Autodesk Fusion 360 part; units mm, degrees
(part 18 of 40)
  spline S39 degree 5 poles (-5.6951, -60.7685) (-5.6979, -60.7993) (-5.7029, -60.8609) (-5.7078, -60.9533) (-5.7097, -61.0766) (-5.7056, -61.231) (-5.6969, -61.3856) (-5.6854, -61.5403) (-5.6723, -61.695) (-5.6583, -61.8498) (-5.6431, -62.0045) (-5.6265, -62.1593) (-5.608, -62.314) (-5.5871, -62.4688) (-5.5641, -62.6235) (-5.539, -62.7782) (-5.5121, -62.9329) (-5.4838, -63.0875) (-5.4542, -63.2421) (-5.4233, -63.3966) (-5.3913, -63.5511) (-5.3579, -63.7055) (-5.3232, -63.8598) (-5.2871, -64.014) (-5.2497, -64.1682) (-5.2109, -64.3222) (-5.1709, -64.4762) (-5.1297, -64.6301) (-5.0873, -64.7839) (-5.0439, -64.9376) (-4.9993, -65.0912) (-4.9536, -65.2447) (-4.9068, -65.398) (-4.8589, -65.5513) (-4.8099, -65.7044) (-4.7599, -65.8574) (-4.7087, -66.0103) (-4.6566, -66.1631) (-4.6035, -66.3158) (-4.5493, -66.4683) (-4.4942, -66.6206) (-4.438, -66.7729) (-4.381, -66.925) (-4.3229, -67.077) (-4.2639, -67.2288) (-4.2039, -67.3804) (-4.143, -67.532) (-4.0812, -67.6833) (-4.0185, -67.8345) (-3.9548, -67.9856) (-3.8903, -68.1365) (-3.8249, -68.2872) (-3.7585, -68.4378) (-3.6913, -68.5882) (-3.6233, -68.7384) (-3.5543, -68.8885) (-3.4846, -69.0384) (-3.4139, -69.1881) (-3.3425, -69.3376) (-3.2701, -69.487) (-3.197, -69.6362) (-3.123, -69.7852) (-3.0482, -69.934) (-2.9726, -70.0826) (-2.8962, -70.2311) (-2.819, -70.3793) (-2.741, -70.5274) (-2.6622, -70.6752) (-2.5826, -70.8229) (-2.5023, -70.9703) (-2.4211, -71.1176) (-2.3556, -71.2352) (-2.3061, -71.3234) (-2.2729, -71.3821) (-2.2563, -71.4115) knots 0 0 0 0 0 0 0.01428571 0.02857143 0.04285714 0.05714286 0.07142857 0.08571429 0.1 0.11428571 0.12857143 0.14285714 0.15714286 0.17142857 0.18571429 0.2 0.21428571 0.22857143 0.24285714 0.25714286 0.27142857 0.28571429 0.3 0.31428571 0.32857143 0.34285714 0.35714286 0.37142857 0.38571429 0.4 0.41428571 0.42857143 0.44285714 0.45714286 0.47142857 0.48571429 0.5 0.51428571 0.52857143 0.54285714 0.55714286 0.57142857 0.58571429 0.6 0.61428571 0.62857143 0.64285714 0.65714286 0.67142857 0.68571429 0.7 0.71428571 0.72857143 0.74285714 0.75714286 0.77142857 0.78571429 0.8 0.81428571 0.82857143 0.84285714 0.85714286 0.87142857 0.88571429 0.9 0.91428571 0.92857143 0.94285714 0.95714286 0.97142857 0.98571429 1 1 1 1 1 1
  line L39 (-5.5428, -59.1442) -> (-5.6951, -60.7685)
  arc A78 (-5.5428, -59.1442) -> (-7.2806, -56.9737) centre (-7.5341, -58.9575) ccw
  arc A79 (-10.6816, -56.435) -> (-7.2806, -56.9737) centre (0, 0) ccw
  arc A80 (-27.5982, -50.3721) -> (-24.5301, -51.9354) centre (0, 0) ccw
  line L40 (24.1948, -56.0345) -> (24.2071, -56.0628) construction
  line L41 (24.2071, -56.0628) -> (24.2308, -56.1198) construction
  line L42 (24.2308, -56.1198) -> (24.264, -56.2062) construction
  line L43 (24.264, -56.2062) -> (24.3039, -56.3229) construction
  line L44 (24.3039, -56.3229) -> (24.3478, -56.4711) construction
  line L45 (24.3478, -56.4711) -> (24.3873, -56.6208) construction
  line L46 (24.3873, -56.6208) -> (24.4241, -56.7714) construction
  line L47 (24.4241, -56.7714) -> (24.4595, -56.9226) construction
  line L48 (24.4595, -56.9226) -> (24.494, -57.0741) construction
  line L49 (24.494, -57.0741) -> (24.5274, -57.226) construction
  line L50 (24.5274, -57.226) -> (24.5594, -57.3783) construction
  line L51 (24.5594, -57.3783) -> (24.5896, -57.5312) construction
  line L52 (24.5896, -57.5312) -> (24.6176, -57.6848) construction
  line L53 (24.6176, -57.6848) -> (24.6435, -57.8391) construction
  line L54 (24.6435, -57.8391) -> (24.6674, -57.994) construction
  line L55 (24.6674, -57.994) -> (24.6897, -58.1494) construction
  line L56 (24.6897, -58.1494) -> (24.7105, -58.3052) construction
  line L57 (24.7105, -58.3052) -> (24.7301, -58.4614) construction
  line L58 (24.7301, -58.4614) -> (24.7485, -58.6179) construction
  line L59 (24.7485, -58.6179) -> (24.7658, -58.7747) construction
  line L60 (24.7658, -58.7747) -> (24.7818, -58.9318) construction
  line L61 (24.7818, -58.9318) -> (24.7965, -59.0893) construction
  line L62 (24.7965, -59.0893) -> (24.8098, -59.2471) construction
  line L63 (24.8098, -59.2471) -> (24.8218, -59.4053) construction
  line L64 (24.8218, -59.4053) -> (24.8325, -59.5638) construction
  line L65 (24.8325, -59.5638) -> (24.842, -59.7226) construction
  line L66 (24.842, -59.7226) -> (24.8504, -59.8817) construction
  line L67 (24.8504, -59.8817) -> (24.8577, -60.0411) construction
  line L68 (24.8577, -60.0411) -> (24.8638, -60.2007) construction
  line L69 (24.8638, -60.2007) -> (24.8689, -60.3605) construction
  line L70 (24.8689, -60.3605) -> (24.8729, -60.5206) construction
  line L71 (24.8729, -60.5206) -> (24.8757, -60.6809) construction
  line L72 (24.8757, -60.6809) -> (24.8776, -60.8415) construction
  line L73 (24.8776, -60.8415) -> (24.8783, -61.0023) construction
  line L74 (24.8783, -61.0023) -> (24.878, -61.1633) construction
  line L75 (24.878, -61.1633) -> (24.8766, -61.3245) construction
  line L76 (24.8766, -61.3245) -> (24.8742, -61.4859) construction
  line L77 (24.8742, -61.4859) -> (24.8708, -61.6475) construction
  line L78 (24.8708, -61.6475) -> (24.8665, -61.8093) construction
  line L79 (24.8665, -61.8093) -> (24.8611, -61.9712) construction
  line L80 (24.8611, -61.9712) -> (24.8548, -62.1334) construction
  line L81 (24.8548, -62.1334) -> (24.8475, -62.2957) construction
  line L82 (24.8475, -62.2957) -> (24.8392, -62.4581) construction
  line L83 (24.8392, -62.4581) -> (24.83, -62.6207) construction
  line L84 (24.83, -62.6207) -> (24.8199, -62.7835) construction
  line L85 (24.8199, -62.7835) -> (24.8088, -62.9464) construction
  line L86 (24.8088, -62.9464) -> (24.7967, -63.1095) construction
  line L87 (24.7967, -63.1095) -> (24.7838, -63.2727) construction
  line L88 (24.7838, -63.2727) -> (24.77, -63.436) construction
  line L89 (24.77, -63.436) -> (24.7552, -63.5995) construction
  line L90 (24.7552, -63.5995) -> (24.7396, -63.7631) construction
  line L91 (24.7396, -63.7631) -> (24.723, -63.9268) construction
  line L92 (24.723, -63.9268) -> (24.7056, -64.0906) construction
  line L93 (24.7056, -64.0906) -> (24.6873, -64.2545) construction
  line L94 (24.6873, -64.2545) -> (24.6681, -64.4185) construction
  line L95 (24.6681, -64.4185) -> (24.648, -64.5826) construction
  line L96 (24.648, -64.5826) -> (24.6271, -64.7468) construction
  line L97 (24.6271, -64.7468) -> (24.6054, -64.9111) construction
  line L98 (24.6054, -64.9111) -> (24.5828, -65.0755) construction
  line L99 (24.5828, -65.0755) -> (24.5593, -65.24) construction
  line L100 (24.5593, -65.24) -> (24.535, -65.4046) construction
  line L101 (24.535, -65.4046) -> (24.5098, -65.5692) construction
  line L102 (24.5098, -65.5692) -> (24.4839, -65.734) construction
  line L103 (24.4839, -65.734) -> (24.4571, -65.8987) construction
  line L104 (24.4571, -65.8987) -> (24.4294, -66.0636) construction
  line L105 (24.4294, -66.0636) -> (24.401, -66.2285) construction
  line L106 (24.401, -66.2285) -> (24.3718, -66.3935) construction
  line L107 (24.3718, -66.3935) -> (24.3417, -66.5585) construction
  line L108 (24.3417, -66.5585) -> (24.3108, -66.7236) construction
  line L109 (24.3108, -66.7236) -> (24.2792, -66.8887) construction
  line L110 (24.2792, -66.8887) -> (24.2532, -67.0208) construction
  line L111 (24.2532, -67.0208) -> (24.2334, -67.1199) construction
  line L112 (24.2334, -67.1199) -> (24.22, -67.186) construction
  line L113 (24.22, -67.186) -> (24.2132, -67.2191) construction
  line L114 (60.7685, -5.6951) -> (60.7993, -5.6979) construction
  line L115 (60.7993, -5.6979) -> (60.8609, -5.7029) construction
  line L116 (60.8609, -5.7029) -> (60.9533, -5.7078) construction
  line L117 (60.9533, -5.7078) -> (61.0766, -5.7097) construction
  line L118 (61.0766, -5.7097) -> (61.231, -5.7056) construction
  line L119 (61.231, -5.7056) -> (61.3856, -5.6969) construction
  line L120 (61.3856, -5.6969) -> (61.5403, -5.6854) construction
  line L121 (61.5403, -5.6854) -> (61.695, -5.6723) construction
  line L122 (61.695, -5.6723) -> (61.8498, -5.6583) construction
  line L123 (61.8498, -5.6583) -> (62.0045, -5.6431) construction
  line L124 (62.0045, -5.6431) -> (62.1593, -5.6265) construction
  line L125 (62.1593, -5.6265) -> (62.314, -5.608) construction
  line L126 (62.314, -5.608) -> (62.4688, -5.5871) construction
  line L127 (62.4688, -5.5871) -> (62.6235, -5.5641) construction
  line L128 (62.6235, -5.5641) -> (62.7782, -5.539) construction
  line L129 (62.7782, -5.539) -> (62.9329, -5.5121) construction
  line L130 (62.9329, -5.5121) -> (63.0875, -5.4838) construction
  line L131 (63.0875, -5.4838) -> (63.2421, -5.4542) construction
  line L132 (63.2421, -5.4542) -> (63.3966, -5.4233) construction
  line L133 (63.3966, -5.4233) -> (63.5511, -5.3913) construction
  line L134 (63.5511, -5.3913) -> (63.7055, -5.3579) construction
  line L135 (63.7055, -5.3579) -> (63.8598, -5.3232) construction
  line L136 (63.8598, -5.3232) -> (64.014, -5.2871) construction
  line L137 (64.014, -5.2871) -> (64.1682, -5.2497) construction
  line L138 (64.1682, -5.2497) -> (64.3222, -5.2109) construction
  line L139 (64.3222, -5.2109) -> (64.4762, -5.1709) construction
  line L140 (64.4762, -5.1709) -> (64.6301, -5.1297) construction
  line L141 (64.6301, -5.1297) -> (64.7839, -5.0873) construction
  line L142 (64.7839, -5.0873) -> (64.9376, -5.0439) construction
  line L143 (64.9376, -5.0439) -> (65.0912, -4.9993) construction
  line L144 (65.0912, -4.9993) -> (65.2447, -4.9536) construction
  line L145 (65.2447, -4.9536) -> (65.398, -4.9068) construction
  line L146 (65.398, -4.9068) -> (65.5513, -4.8589) construction
  line L147 (65.5513, -4.8589) -> (65.7044, -4.8099) construction
  line L148 (65.7044, -4.8099) -> (65.8574, -4.7599) construction
  line L149 (65.8574, -4.7599) -> (66.0103, -4.7087) construction
  line L150 (66.0103, -4.7087) -> (66.1631, -4.6566) construction
  line L151 (66.1631, -4.6566) -> (66.3158, -4.6035) construction
  line L152 (66.3158, -4.6035) -> (66.4683, -4.5493) construction
  line L153 (66.4683, -4.5493) -> (66.6206, -4.4942) construction
  line L154 (66.6206, -4.4942) -> (66.7729, -4.438) construction
  line L155 (66.7729, -4.438) -> (66.925, -4.381) construction
  line L156 (66.925, -4.381) -> (67.077, -4.3229) construction
  line L157 (67.077, -4.3229) -> (67.2288, -4.2639) construction
  line L158 (67.2288, -4.2639) -> (67.3804, -4.2039) construction
  line L159 (67.3804, -4.2039) -> (67.532, -4.143) construction
  line L160 (67.532, -4.143) -> (67.6833, -4.0812) construction
  line L161 (67.6833, -4.0812) -> (67.8345, -4.0185) construction
  line L162 (67.8345, -4.0185) -> (67.9856, -3.9548) construction
  line L163 (67.9856, -3.9548) -> (68.1365, -3.8903) construction
  line L164 (68.1365, -3.8903) -> (68.2872, -3.8249) construction
  line L165 (68.2872, -3.8249) -> (68.4378, -3.7585) construction
  line L166 (68.4378, -3.7585) -> (68.5882, -3.6913) construction
  line L167 (68.5882, -3.6913) -> (68.7384, -3.6233) construction
  line L168 (68.7384, -3.6233) -> (68.8885, -3.5543) construction
  line L169 (68.8885, -3.5543) -> (69.0384, -3.4846) construction
  line L170 (69.0384, -3.4846) -> (69.1881, -3.4139) construction
  line L171 (69.1881, -3.4139) -> (69.3376, -3.3425) construction
  line L172 (69.3376, -3.3425) -> (69.487, -3.2701) construction
  line L173 (69.487, -3.2701) -> (69.6362, -3.197) construction
  line L174 (69.6362, -3.197) -> (69.7852, -3.123) construction
  line L175 (69.7852, -3.123) -> (69.934, -3.0482) construction
  line L176 (69.934, -3.0482) -> (70.0826, -2.9726) construction
  line L177 (70.0826, -2.9726) -> (70.2311, -2.8962) construction
  line L178 (70.2311, -2.8962) -> (70.3793, -2.819) construction
  line L179 (70.3793, -2.819) -> (70.5274, -2.741) construction
  line L180 (70.5274, -2.741) -> (70.6752, -2.6622) construction
  line L181 (70.6752, -2.6622) -> (70.8229, -2.5826) construction
  line L182 (70.8229, -2.5826) -> (70.9703, -2.5023) construction
  line L183 (70.9703, -2.5023) -> (71.1176, -2.4211) construction
  line L184 (71.1176, -2.4211) -> (71.2352, -2.3556) construction
  line L185 (71.2352, -2.3556) -> (71.3234, -2.3061) construction
  line L186 (71.3234, -2.3061) -> (71.3821, -2.2729) construction
  line L187 (71.3821, -2.2729) -> (71.4115, -2.2563) construction
  line L188 (-45.8153, -40.3263) -> (-45.8385, -40.3467) construction
  line L189 (-45.8385, -40.3467) -> (-45.8854, -40.3868) construction
  line L190 (-45.8854, -40.3868) -> (-45.9573, -40.4451) construction
  line L191 (-45.9573, -40.4451) -> (-46.056, -40.5192) construction
  line L192 (-46.056, -40.5192) -> (-46.1833, -40.6066) construction
  line L193 (-46.1833, -40.6066) -> (-46.3135, -40.6904) construction
  line L194 (-46.3135, -40.6904) -> (-46.4454, -40.772) construction
  line L195 (-46.4454, -40.772) -> (-46.5782, -40.8524) construction
  line L196 (-46.5782, -40.8524) -> (-46.7117, -40.932) construction
  line L197 (-46.7117, -40.932) -> (-46.8458, -41.0107) construction
  line L198 (-46.8458, -41.0107) -> (-46.9807, -41.0883) construction
  line L199 (-46.9807, -41.0883) -> (-47.1168, -41.1642) construction
  line L200 (-47.1168, -41.1642) -> (-47.2543, -41.2383) construction
  line L201 (-47.2543, -41.2383) -> (-47.393, -41.3106) construction
  line L202 (-47.393, -41.3106) -> (-47.5329, -41.3813) construction
  line L203 (-47.5329, -41.3813) -> (-47.6738, -41.4504) construction
  line L204 (-47.6738, -41.4504) -> (-47.8156, -41.5184) construction
  line L205 (-47.8156, -41.5184) -> (-47.9581, -41.5853) construction
  line L206 (-47.9581, -41.5853) -> (-48.1012, -41.6512) construction
  line L207 (-48.1012, -41.6512) -> (-48.245, -41.716) construction
  line L208 (-48.245, -41.716) -> (-48.3895, -41.7798) construction
  line L209 (-48.3895, -41.7798) -> (-48.5347, -41.8424) construction
  line L210 (-48.5347, -41.8424) -> (-48.6807, -41.9039) construction
  line L211 (-48.6807, -41.9039) -> (-48.8274, -41.9642) construction
  line L212 (-48.8274, -41.9642) -> (-48.9749, -42.0234) construction
  line L213 (-48.9749, -42.0234) -> (-49.123, -42.0815) construction
  line L214 (-49.123, -42.0815) -> (-49.2717, -42.1386) construction
  line L215 (-49.2717, -42.1386) -> (-49.421, -42.1947) construction
  line L216 (-49.421, -42.1947) -> (-49.5709, -42.2499) construction
  line L217 (-49.5709, -42.2499) -> (-49.7214, -42.3041) construction
  line L218 (-49.7214, -42.3041) -> (-49.8724, -42.3574) construction
  line L219 (-49.8724, -42.3574) -> (-50.024, -42.4097) construction
  line L220 (-50.024, -42.4097) -> (-50.1761, -42.461) construction
  line L221 (-50.1761, -42.461) -> (-50.3288, -42.5114) construction
  line L222 (-50.3288, -42.5114) -> (-50.482, -42.5608) construction
  line L223 (-50.482, -42.5608) -> (-50.6358, -42.6094) construction
  line L224 (-50.6358, -42.6094) -> (-50.79, -42.657) construction
  line L225 (-50.79, -42.657) -> (-50.9447, -42.7037) construction
  line L226 (-50.9447, -42.7037) -> (-51.0999, -42.7495) construction
  line L227 (-51.0999, -42.7495) -> (-51.2556, -42.7945) construction
  line L228 (-51.2556, -42.7945) -> (-51.4118, -42.8386) construction
  line L229 (-51.4118, -42.8386) -> (-51.5684, -42.8818) construction
  line L230 (-51.5684, -42.8818) -> (-51.7255, -42.9241) construction
  line L231 (-51.7255, -42.9241) -> (-51.883, -42.9656) construction
  line L232 (-51.883, -42.9656) -> (-52.0409, -43.0063) construction
  line L233 (-52.0409, -43.0063) -> (-52.1993, -43.0461) construction
  line L234 (-52.1993, -43.0461) -> (-52.3581, -43.085) construction
  line L235 (-52.3581, -43.085) -> (-52.5173, -43.1231) construction
  line L236 (-52.5173, -43.1231) -> (-52.6769, -43.1604) construction
  line L237 (-52.6769, -43.1604) -> (-52.8369, -43.1969) construction
  line L238 (-52.8369, -43.1969) -> (-52.9973, -43.2326) construction
  line L239 (-52.9973, -43.2326) -> (-53.1581, -43.2674) construction
  line L240 (-53.1581, -43.2674) -> (-53.3193, -43.3015) construction
  line L241 (-53.3193, -43.3015) -> (-53.4809, -43.3347) construction
  line L242 (-53.4809, -43.3347) -> (-53.6428, -43.3672) construction
  line L243 (-53.6428, -43.3672) -> (-53.8051, -43.3988) construction
  line L244 (-53.8051, -43.3988) -> (-53.9677, -43.4297) construction
  line L245 (-53.9677, -43.4297) -> (-54.1307, -43.4597) construction
  line L246 (-54.1307, -43.4597) -> (-54.294, -43.489) construction
  line L247 (-54.294, -43.489) -> (-54.4577, -43.5175) construction
  line L248 (-54.4577, -43.5175) -> (-54.6217, -43.5453) construction
  line L249 (-54.6217, -43.5453) -> (-54.7861, -43.5723) construction
  line L250 (-54.7861, -43.5723) -> (-54.9508, -43.5984) construction
  line L251 (-54.9508, -43.5984) -> (-55.1158, -43.6239) construction
  line L252 (-55.1158, -43.6239) -> (-55.2811, -43.6486) construction
  line L253 (-55.2811, -43.6486) -> (-55.4467, -43.6725) construction
  line L254 (-55.4467, -43.6725) -> (-55.6126, -43.6956) construction
  line L255 (-55.6126, -43.6956) -> (-55.7789, -43.718) construction
  line L256 (-55.7789, -43.718) -> (-55.9454, -43.7397) construction
  line L257 (-55.9454, -43.7397) -> (-56.1122, -43.7606) construction
  line L258 (-56.1122, -43.7606) -> (-56.2459, -43.7767) construction
  line L259 (-56.2459, -43.7767) -> (-56.3463, -43.7885) construction
  line L260 (-56.3463, -43.7885) -> (-56.4133, -43.7962) construction
  line L261 (-56.4133, -43.7962) -> (-56.4469, -43.8) construction
  line L262 (45.8153, -40.3263) -> (45.8385, -40.3467) construction
  line L263 (45.8385, -40.3467) -> (45.8854, -40.3868) construction
  line L264 (45.8854, -40.3868) -> (45.9573, -40.4451) construction
  line L265 (45.9573, -40.4451) -> (46.056, -40.5192) construction
  line L266 (46.056, -40.5192) -> (46.1833, -40.6066) construction
  line L267 (46.1833, -40.6066) -> (46.3135, -40.6904) construction
  line L268 (46.3135, -40.6904) -> (46.4454, -40.772) construction
  line L269 (46.4454, -40.772) -> (46.5782, -40.8524) construction
  line L270 (46.5782, -40.8524) -> (46.7117, -40.932) construction
  line L271 (46.7117, -40.932) -> (46.8458, -41.0107) construction
  line L272 (46.8458, -41.0107) -> (46.9807, -41.0883) construction
  line L273 (46.9807, -41.0883) -> (47.1168, -41.1642) construction
  line L274 (47.1168, -41.1642) -> (47.2543, -41.2383) construction
  line L275 (47.2543, -41.2383) -> (47.393, -41.3106) construction
  line L276 (47.393, -41.3106) -> (47.5329, -41.3813) construction
  line L277 (47.5329, -41.3813) -> (47.6738, -41.4504) construction
  line L278 (47.6738, -41.4504) -> (47.8156, -41.5184) construction
  line L279 (47.8156, -41.5184) -> (47.9581, -41.5853) construction
  line L280 (47.9581, -41.5853) -> (48.1012, -41.6512) construction
  line L281 (48.1012, -41.6512) -> (48.245, -41.716) construction
  line L282 (48.245, -41.716) -> (48.3895, -41.7798) construction
  line L283 (48.3895, -41.7798) -> (48.5347, -41.8424) construction
  line L284 (48.5347, -41.8424) -> (48.6807, -41.9039) construction
  line L285 (48.6807, -41.9039) -> (48.8274, -41.9642) construction
  line L286 (48.8274, -41.9642) -> (48.9749, -42.0234) construction
  line L287 (48.9749, -42.0234) -> (49.123, -42.0815) construction
  line L288 (49.123, -42.0815) -> (49.2717, -42.1386) construction
  line L289 (49.2717, -42.1386) -> (49.421, -42.1947) construction
  line L290 (49.421, -42.1947) -> (49.5709, -42.2499) construction
  line L291 (49.5709, -42.2499) -> (49.7214, -42.3041) construction
  line L292 (49.7214, -42.3041) -> (49.8724, -42.3574) construction
  line L293 (49.8724, -42.3574) -> (50.024, -42.4097) construction
  line L294 (50.024, -42.4097) -> (50.1761, -42.461) construction
  line L295 (50.1761, -42.461) -> (50.3288, -42.5114) construction
  line L296 (50.3288, -42.5114) -> (50.482, -42.5608) construction
  line L297 (50.482, -42.5608) -> (50.6358, -42.6094) construction
  line L298 (50.6358, -42.6094) -> (50.79, -42.657) construction
  line L299 (50.79, -42.657) -> (50.9447, -42.7037) construction
  line L300 (50.9447, -42.7037) -> (51.0999, -42.7495) construction
  line L301 (51.0999, -42.7495) -> (51.2556, -42.7945) construction
  line L302 (51.2556, -42.7945) -> (51.4118, -42.8386) construction
  line L303 (51.4118, -42.8386) -> (51.5684, -42.8818) construction
  line L304 (51.5684, -42.8818) -> (51.7255, -42.9241) construction
  line L305 (51.7255, -42.9241) -> (51.883, -42.9656) construction
  line L306 (51.883, -42.9656) -> (52.0409, -43.0063) construction
  line L307 (52.0409, -43.0063) -> (52.1993, -43.0461) construction
  line L308 (52.1993, -43.0461) -> (52.3581, -43.085) construction
  line L309 (52.3581, -43.085) -> (52.5173, -43.1231) construction
  line L310 (52.5173, -43.1231) -> (52.6769, -43.1604) construction
  line L311 (52.6769, -43.1604) -> (52.8369, -43.1969) construction
  line L312 (52.8369, -43.1969) -> (52.9973, -43.2326) construction
  line L313 (52.9973, -43.2326) -> (53.1581, -43.2674) construction
  line L314 (53.1581, -43.2674) -> (53.3193, -43.3015) construction
  line L315 (53.3193, -43.3015) -> (53.4809, -43.3347) construction
  line L316 (53.4809, -43.3347) -> (53.6428, -43.3672) construction
  line L317 (53.6428, -43.3672) -> (53.8051, -43.3988) construction
  line L318 (53.8051, -43.3988) -> (53.9677, -43.4297) construction
  line L319 (53.9677, -43.4297) -> (54.1307, -43.4597) construction
  line L320 (54.1307, -43.4597) -> (54.294, -43.489) construction
  line L321 (54.294, -43.489) -> (54.4577, -43.5175) construction
  line L322 (54.4577, -43.5175) -> (54.6217, -43.5453) construction
  line L323 (54.6217, -43.5453) -> (54.7861, -43.5723) construction
  line L324 (54.7861, -43.5723) -> (54.9508, -43.5984) construction
  line L325 (54.9508, -43.5984) -> (55.1158, -43.6239) construction
  line L326 (55.1158, -43.6239) -> (55.2811, -43.6486) construction
  line L327 (55.2811, -43.6486) -> (55.4467, -43.6725) construction
  line L328 (55.4467, -43.6725) -> (55.6126, -43.6956) construction
  line L329 (55.6126, -43.6956) -> (55.7789, -43.718) construction
  line L330 (55.7789, -43.718) -> (55.9454, -43.7397) construction
  line L331 (55.9454, -43.7397) -> (56.1122, -43.7606) construction
  line L332 (56.1122, -43.7606) -> (56.2459, -43.7767) construction
  line L333 (56.2459, -43.7767) -> (56.3463, -43.7885) construction
  line L334 (56.3463, -43.7885) -> (56.4133, -43.7962) construction
  line L335 (56.4133, -43.7962) -> (56.4469, -43.8) construction
  line L336 (31.1115, -52.5103) -> (31.1272, -52.5368) construction
  line L337 (31.1272, -52.5368) -> (31.1594, -52.5895) construction
  line L338 (31.1594, -52.5895) -> (31.2097, -52.6672) construction
  line L339 (31.2097, -52.6672) -> (31.2807, -52.7681) construction
  line L340 (31.2807, -52.7681) -> (31.3748, -52.8906) construction
  line L341 (31.3748, -52.8906) -> (31.4727, -53.0106) construction
  line L342 (31.4727, -53.0106) -> (31.5729, -53.1289) construction
  line L343 (31.5729, -53.1289) -> (31.6744, -53.2464) construction
  line L344 (31.6744, -53.2464) -> (31.7767, -53.3634) construction
  line L345 (31.7767, -53.3634) -> (31.88, -53.4797) construction
  line L346 (31.88, -53.4797) -> (31.9844, -53.5951) construction
  line L347 (31.9844, -53.5951) -> (32.0903, -53.7094) construction
  line L348 (32.0903, -53.7094) -> (32.1981, -53.8224) construction
  line L349 (32.1981, -53.8224) -> (32.3077, -53.934) construction
  line L350 (32.3077, -53.934) -> (32.419, -54.0444) construction
  line L351 (32.419, -54.0444) -> (32.5316, -54.1537) construction
  line L352 (32.5316, -54.1537) -> (32.6455, -54.2622) construction
  line L353 (32.6455, -54.2622) -> (32.7603, -54.3698) construction
  line L354 (32.7603, -54.3698) -> (32.876, -54.4767) construction
  line L355 (32.876, -54.4767) -> (32.9927, -54.5828) construction
  line L356 (32.9927, -54.5828) -> (33.1105, -54.6881) construction
  line L357 (33.1105, -54.6881) -> (33.2292, -54.7926) construction
  line L358 (33.2292, -54.7926) -> (33.3491, -54.8961) construction
  line L359 (33.3491, -54.8961) -> (33.47, -54.9988) construction
  line L360 (33.47, -54.9988) -> (33.5919, -55.1007) construction
  line L361 (33.5919, -55.1007) -> (33.7148, -55.2017) construction
  line L362 (33.7148, -55.2017) -> (33.8386, -55.302) construction
  line L363 (33.8386, -55.302) -> (33.9633, -55.4015) construction
  line L364 (33.9633, -55.4015) -> (34.0888, -55.5003) construction
  line L365 (34.0888, -55.5003) -> (34.2151, -55.5984) construction
  line L366 (34.2151, -55.5984) -> (34.3423, -55.6957) construction
  line L367 (34.3423, -55.6957) -> (34.4703, -55.7923) construction
  line L368 (34.4703, -55.7923) -> (34.5991, -55.8881) construction
  line L369 (34.5991, -55.8881) -> (34.7288, -55.9832) construction
  line L370 (34.7288, -55.9832) -> (34.8592, -56.0776) construction
  line L371 (34.8592, -56.0776) -> (34.9905, -56.1712) construction
  line L372 (34.9905, -56.1712) -> (35.1224, -56.2642) construction
  line L373 (35.1224, -56.2642) -> (35.2552, -56.3564) construction
  line L374 (35.2552, -56.3564) -> (35.3886, -56.448) construction
  line L375 (35.3886, -56.448) -> (35.5228, -56.5388) construction
  line L376 (35.5228, -56.5388) -> (35.6577, -56.629) construction
  line L377 (35.6577, -56.629) -> (35.7933, -56.7185) construction
  line L378 (35.7933, -56.7185) -> (35.9295, -56.8073) construction
  line L379 (35.9295, -56.8073) -> (36.0665, -56.8955) construction
  line L380 (36.0665, -56.8955) -> (36.2042, -56.9829) construction
  line L381 (36.2042, -56.9829) -> (36.3425, -57.0697) construction
  line L382 (36.3425, -57.0697) -> (36.4815, -57.1558) construction
  line L383 (36.4815, -57.1558) -> (36.6211, -57.2413) construction
  line L384 (36.6211, -57.2413) -> (36.7614, -57.3261) construction
  line L385 (36.7614, -57.3261) -> (36.9023, -57.4102) construction
  line L386 (36.9023, -57.4102) -> (37.0438, -57.4937) construction
  line L387 (37.0438, -57.4937) -> (37.186, -57.5765) construction
  line L388 (37.186, -57.5765) -> (37.3288, -57.6587) construction
  line L389 (37.3288, -57.6587) -> (37.4721, -57.7403) construction
  line L390 (37.4721, -57.7403) -> (37.6161, -57.8212) construction
  line L391 (37.6161, -57.8212) -> (37.7607, -57.9014) construction
  line L392 (37.7607, -57.9014) -> (37.9058, -57.981) construction
  line L393 (37.9058, -57.981) -> (38.0515, -58.06) construction
  line L394 (38.0515, -58.06) -> (38.1978, -58.1383) construction
  line L395 (38.1978, -58.1383) -> (38.3447, -58.216) construction
  line L396 (38.3447, -58.216) -> (38.4921, -58.2931) construction
  line L397 (38.4921, -58.2931) -> (38.6401, -58.3695) construction
  line L398 (38.6401, -58.3695) -> (38.7886, -58.4453) construction
  line L399 (38.7886, -58.4453) -> (38.9377, -58.5205) construction
  line L400 (38.9377, -58.5205) -> (39.0873, -58.595) construction
  line L401 (39.0873, -58.595) -> (39.2374, -58.669) construction
  line L402 (39.2374, -58.669) -> (39.3881, -58.7423) construction
  line L403 (39.3881, -58.7423) -> (39.5393, -58.8149) construction
  line L404 (39.5393, -58.8149) -> (39.6909, -58.887) construction
  line L405 (39.6909, -58.887) -> (39.8431, -58.9584) construction
  line L406 (39.8431, -58.9584) -> (39.9653, -59.0151) construction
  line L407 (39.9653, -59.0151) -> (40.0572, -59.0573) construction
  line L408 (40.0572, -59.0573) -> (40.1185, -59.0853) construction
  line L409 (40.1185, -59.0853) -> (40.1492, -59.0993) construction
  line L410 (5.6951, -60.7685) -> (5.6979, -60.7993) construction
  line L411 (5.6979, -60.7993) -> (5.7029, -60.8609) construction
  line L412 (5.7029, -60.8609) -> (5.7078, -60.9533) construction
  line L413 (5.7078, -60.9533) -> (5.7097, -61.0766) construction
  line L414 (5.7097, -61.0766) -> (5.7056, -61.231) construction
  line L415 (5.7056, -61.231) -> (5.6969, -61.3856) construction
  line L416 (5.6969, -61.3856) -> (5.6854, -61.5403) construction
  line L417 (5.6854, -61.5403) -> (5.6723, -61.695) construction
  line L418 (5.6723, -61.695) -> (5.6583, -61.8498) construction
  line L419 (5.6583, -61.8498) -> (5.6431, -62.0045) construction
  line L420 (5.6431, -62.0045) -> (5.6265, -62.1593) construction
  line L421 (5.6265, -62.1593) -> (5.608, -62.314) construction
  line L422 (5.608, -62.314) -> (5.5871, -62.4688) construction
  line L423 (5.5871, -62.4688) -> (5.5641, -62.6235) construction
  line L424 (5.5641, -62.6235) -> (5.539, -62.7782) construction
  line L425 (5.539, -62.7782) -> (5.5121, -62.9329) construction
  line L426 (5.5121, -62.9329) -> (5.4838, -63.0875) construction
  line L427 (5.4838, -63.0875) -> (5.4542, -63.2421) construction
  line L428 (5.4542, -63.2421) -> (5.4233, -63.3966) construction
  line L429 (5.4233, -63.3966) -> (5.3913, -63.5511) construction
  line L430 (5.3913, -63.5511) -> (5.3579, -63.7055) construction
  line L431 (5.3579, -63.7055) -> (5.3232, -63.8598) construction
  line L432 (5.3232, -63.8598) -> (5.2871, -64.014) construction
  line L433 (5.2871, -64.014) -> (5.2497, -64.1682) construction
  line L434 (5.2497, -64.1682) -> (5.2109, -64.3222) construction
  line L435 (5.2109, -64.3222) -> (5.1709, -64.4762) construction
  line L436 (5.1709, -64.4762) -> (5.1297, -64.6301) construction
  line L437 (5.1297, -64.6301) -> (5.0873, -64.7839) construction
  line L438 (5.0873, -64.7839) -> (5.0439, -64.9376) construction
  line L439 (5.0439, -64.9376) -> (4.9993, -65.0912) construction
  line L440 (4.9993, -65.0912) -> (4.9536, -65.2447) construction
  line L441 (4.9536, -65.2447) -> (4.9068, -65.398) construction
  line L442 (4.9068, -65.398) -> (4.8589, -65.5513) construction
  line L443 (4.8589, -65.5513) -> (4.8099, -65.7044) construction
  line L444 (4.8099, -65.7044) -> (4.7599, -65.8574) construction
  line L445 (4.7599, -65.8574) -> (4.7087, -66.0103) construction
  line L446 (4.7087, -66.0103) -> (4.6566, -66.1631) construction
  line L447 (4.6566, -66.1631) -> (4.6035, -66.3158) construction
  line L448 (4.6035, -66.3158) -> (4.5493, -66.4683) construction
  line L449 (4.5493, -66.4683) -> (4.4942, -66.6206) construction
  line L450 (4.4942, -66.6206) -> (4.438, -66.7729) construction
  line L451 (4.438, -66.7729) -> (4.381, -66.925) construction
  line L452 (4.381, -66.925) -> (4.3229, -67.077) construction
  line L453 (4.3229, -67.077) -> (4.2639, -67.2288) construction
  line L454 (4.2639, -67.2288) -> (4.2039, -67.3804) construction
  line L455 (4.2039, -67.3804) -> (4.143, -67.532) construction
  line L456 (4.143, -67.532) -> (4.0812, -67.6833) construction
  line L457 (4.0812, -67.6833) -> (4.0185, -67.8345) construction
  line L458 (4.0185, -67.8345) -> (3.9548, -67.9856) construction
  line L459 (3.9548, -67.9856) -> (3.8903, -68.1365) construction
  line L460 (3.8903, -68.1365) -> (3.8249, -68.2872) construction
  line L461 (3.8249, -68.2872) -> (3.7585, -68.4378) construction
  line L462 (3.7585, -68.4378) -> (3.6913, -68.5882) construction
  line L463 (3.6913, -68.5882) -> (3.6233, -68.7384) construction
  line L464 (3.6233, -68.7384) -> (3.5543, -68.8885) construction
  line L465 (3.5543, -68.8885) -> (3.4846, -69.0384) construction
  line L466 (3.4846, -69.0384) -> (3.4139, -69.1881) construction
  line L467 (3.4139, -69.1881) -> (3.3425, -69.3376) construction
  line L468 (3.3425, -69.3376) -> (3.2701, -69.487) construction
  line L469 (3.2701, -69.487) -> (3.197, -69.6362) construction
  line L470 (3.197, -69.6362) -> (3.123, -69.7852) construction
  line L471 (3.123, -69.7852) -> (3.0482, -69.934) construction
  line L472 (3.0482, -69.934) -> (2.9726, -70.0826) construction
  line L473 (2.9726, -70.0826) -> (2.8962, -70.2311) construction
  line L474 (2.8962, -70.2311) -> (2.819, -70.3793) construction
  line L475 (2.819, -70.3793) -> (2.741, -70.5274) construction
  line L476 (2.741, -70.5274) -> (2.6622, -70.6752) construction
  line L477 (2.6622, -70.6752) -> (2.5826, -70.8229) construction
  line L478 (2.5826, -70.8229) -> (2.5023, -70.9703) construction
  line L479 (2.5023, -70.9703) -> (2.4211, -71.1176) construction
  line L480 (2.4211, -71.1176) -> (2.3556, -71.2352) construction
  line L481 (2.3556, -71.2352) -> (2.3061, -71.3234) construction
  line L482 (2.3061, -71.3234) -> (2.2729, -71.3821) construction
  line L483 (2.2729, -71.3821) -> (2.2563, -71.4115) construction
  line L484 (-13.3622, 59.5542) -> (-13.369, 59.5843) construction
  line L485 (-13.369, 59.5843) -> (-13.3833, 59.6444) construction
  line L486 (-13.3833, 59.6444) -> (-13.4071, 59.7338) construction
  line L487 (-13.4071, 59.7338) -> (-13.4435, 59.8517) construction
  line L488 (-13.4435, 59.8517) -> (-13.4951, 59.9973) construction
  line L489 (-13.4951, 59.9973) -> (-13.5511, 60.1416) construction
  line L490 (-13.5511, 60.1416) -> (-13.6099, 60.2852) construction
  line L491 (-13.6099, 60.2852) -> (-13.6701, 60.4283) construction
  line L492 (-13.6701, 60.4283) -> (-13.7313, 60.5711) construction
  line L493 (-13.7313, 60.5711) -> (-13.7935, 60.7136) construction
  line L494 (-13.7935, 60.7136) -> (-13.8571, 60.8557) construction
  line L495 (-13.8571, 60.8557) -> (-13.9226, 60.9971) construction
  line L496 (-13.9226, 60.9971) -> (-13.9902, 61.1379) construction
  line L497 (-13.9902, 61.1379) -> (-14.06, 61.2779) construction
  line L498 (-14.06, 61.2779) -> (-14.1316, 61.4173) construction
  line L499 (-14.1316, 61.4173) -> (-14.205, 61.5561) construction
  line L500 (-14.205, 61.5561) -> (-14.2797, 61.6944) construction
  line L501 (-14.2797, 61.6944) -> (-14.3557, 61.8322) construction
  line L502 (-14.3557, 61.8322) -> (-14.4327, 61.9697) construction
  line L503 (-14.4327, 61.9697) -> (-14.5109, 62.1067) construction
  line L504 (-14.5109, 62.1067) -> (-14.5904, 62.2432) construction
  line L505 (-14.5904, 62.2432) -> (-14.6711, 62.3792) construction
  line L506 (-14.6711, 62.3792) -> (-14.753, 62.5148) construction
  line L507 (-14.753, 62.5148) -> (-14.8363, 62.6498) construction
  line L508 (-14.8363, 62.6498) -> (-14.9208, 62.7843) construction
  line L509 (-14.9208, 62.7843) -> (-15.0064, 62.9184) construction
  line L510 (-15.0064, 62.9184) -> (-15.0932, 63.052) construction
  line L511 (-15.0932, 63.052) -> (-15.181, 63.1852) construction
  line L512 (-15.181, 63.1852) -> (-15.2698, 63.318) construction
  line L513 (-15.2698, 63.318) -> (-15.3597, 63.4503) construction
  line L514 (-15.3597, 63.4503) -> (-15.4506, 63.5821) construction
  line L515 (-15.4506, 63.5821) -> (-15.5425, 63.7135) construction
  line L516 (-15.5425, 63.7135) -> (-15.6354, 63.8445) construction
  line L517 (-15.6354, 63.8445) -> (-15.7293, 63.975) construction
  line L518 (-15.7293, 63.975) -> (-15.8242, 64.105) construction
  line L519 (-15.8242, 64.105) -> (-15.92, 64.2346) construction
  line L520 (-15.92, 64.2346) -> (-16.0168, 64.3638) construction
  line L521 (-16.0168, 64.3638) -> (-16.1146, 64.4926) construction
  line L522 (-16.1146, 64.4926) -> (-16.2132, 64.6209) construction
  line L523 (-16.2132, 64.6209) -> (-16.3127, 64.7488) construction
  line L524 (-16.3127, 64.7488) -> (-16.4131, 64.8762) construction
  line L525 (-16.4131, 64.8762) -> (-16.5144, 65.0032) construction
  line L526 (-16.5144, 65.0032) -> (-16.6166, 65.1298) construction
  line L527 (-16.6166, 65.1298) -> (-16.7196, 65.256) construction
  line L528 (-16.7196, 65.256) -> (-16.8235, 65.3817) construction
  line L529 (-16.8235, 65.3817) -> (-16.9283, 65.507) construction
  line L530 (-16.9283, 65.507) -> (-17.0338, 65.6318) construction
  line L531 (-17.0338, 65.6318) -> (-17.1402, 65.7562) construction
  line L532 (-17.1402, 65.7562) -> (-17.2474, 65.8802) construction
  line L533 (-17.2474, 65.8802) -> (-17.3555, 66.0038) construction
  line L534 (-17.3555, 66.0038) -> (-17.4643, 66.1269) construction
  line L535 (-17.4643, 66.1269) -> (-17.5739, 66.2497) construction
  line L536 (-17.5739, 66.2497) -> (-17.6842, 66.3719) construction
  line L537 (-17.6842, 66.3719) -> (-17.7954, 66.4938) construction
  line L538 (-17.7954, 66.4938) -> (-17.9073, 66.6152) construction
  line L539 (-17.9073, 66.6152) -> (-18.02, 66.7362) construction
  line L540 (-18.02, 66.7362) -> (-18.1335, 66.8568) construction
  line L541 (-18.1335, 66.8568) -> (-18.2477, 66.9769) construction
  line L542 (-18.2477, 66.9769) -> (-18.3626, 67.0966) construction
  line L543 (-18.3626, 67.0966) -> (-18.4782, 67.2159) construction
  line L544 (-18.4782, 67.2159) -> (-18.5946, 67.3347) construction
  line L545 (-18.5946, 67.3347) -> (-18.7118, 67.4531) construction
  line L546 (-18.7118, 67.4531) -> (-18.8296, 67.5711) construction
  line L547 (-18.8296, 67.5711) -> (-18.9481, 67.6887) construction
  line L548 (-18.9481, 67.6887) -> (-19.0674, 67.8058) construction
  line L549 (-19.0674, 67.8058) -> (-19.1873, 67.9225) construction
  line L550 (-19.1873, 67.9225) -> (-19.3079, 68.0388) construction
  line L551 (-19.3079, 68.0388) -> (-19.4293, 68.1546) construction
  line L552 (-19.4293, 68.1546) -> (-19.5512, 68.27) construction
  line L553 (-19.5512, 68.27) -> (-19.6739, 68.385) construction
  line L554 (-19.6739, 68.385) -> (-19.7726, 68.4767) construction
  line L555 (-19.7726, 68.4767) -> (-19.8469, 68.5452) construction
  line L556 (-19.8469, 68.5452) -> (-19.8966, 68.5908) construction
  line L557 (-19.8966, 68.5908) -> (-19.9215, 68.6136) construction
  line L558 (24.1948, 56.0345) -> (24.2071, 56.0628) construction
  line L559 (24.2071, 56.0628) -> (24.2308, 56.1198) construction
  line L560 (24.2308, 56.1198) -> (24.264, 56.2062) construction
  line L561 (24.264, 56.2062) -> (24.3039, 56.3229) construction
  line L562 (24.3039, 56.3229) -> (24.3478, 56.4711) construction
  line L563 (24.3478, 56.4711) -> (24.3873, 56.6208) construction
  line L564 (24.3873, 56.6208) -> (24.4241, 56.7714) construction
  line L565 (24.4241, 56.7714) -> (24.4595, 56.9226) construction
  line L566 (24.4595, 56.9226) -> (24.494, 57.0741) construction
  line L567 (24.494, 57.0741) -> (24.5274, 57.226) construction
  line L568 (24.5274, 57.226) -> (24.5594, 57.3783) construction
  line L569 (24.5594, 57.3783) -> (24.5896, 57.5312) construction
  line L570 (24.5896, 57.5312) -> (24.6176, 57.6848) construction
  line L571 (24.6176, 57.6848) -> (24.6435, 57.8391) construction
  line L572 (24.6435, 57.8391) -> (24.6674, 57.994) construction
  line L573 (24.6674, 57.994) -> (24.6897, 58.1494) construction
  line L574 (24.6897, 58.1494) -> (24.7105, 58.3052) construction
  line L575 (24.7105, 58.3052) -> (24.7301, 58.4614) construction
  line L576 (24.7301, 58.4614) -> (24.7485, 58.6179) construction
  line L577 (24.7485, 58.6179) -> (24.7658, 58.7747) construction
  line L578 (24.7658, 58.7747) -> (24.7818, 58.9318) construction
  line L579 (24.7818, 58.9318) -> (24.7965, 59.0893) construction
  line L580 (24.7965, 59.0893) -> (24.8098, 59.2471) construction
  line L581 (24.8098, 59.2471) -> (24.8218, 59.4053) construction
  line L582 (24.8218, 59.4053) -> (24.8325, 59.5638) construction
  line L583 (24.8325, 59.5638) -> (24.842, 59.7226) construction
  line L584 (24.842, 59.7226) -> (24.8504, 59.8817) construction
  line L585 (24.8504, 59.8817) -> (24.8577, 60.0411) construction
  line L586 (24.8577, 60.0411) -> (24.8638, 60.2007) construction
  line L587 (24.8638, 60.2007) -> (24.8689, 60.3605) construction
  line L588 (24.8689, 60.3605) -> (24.8729, 60.5206) construction
  line L589 (24.8729, 60.5206) -> (24.8757, 60.6809) construction
  line L590 (24.8757, 60.6809) -> (24.8776, 60.8415) construction
  line L591 (24.8776, 60.8415) -> (24.8783, 61.0023) construction
  line L592 (24.8783, 61.0023) -> (24.878, 61.1633) construction
  line L593 (24.878, 61.1633) -> (24.8766, 61.3245) construction
  line L594 (24.8766, 61.3245) -> (24.8742, 61.4859) construction
  line L595 (24.8742, 61.4859) -> (24.8708, 61.6475) construction
  line L596 (24.8708, 61.6475) -> (24.8665, 61.8093) construction
  line L597 (24.8665, 61.8093) -> (24.8611, 61.9712) construction
  line L598 (24.8611, 61.9712) -> (24.8548, 62.1334) construction
  line L599 (24.8548, 62.1334) -> (24.8475, 62.2957) construction
  line L600 (24.8475, 62.2957) -> (24.8392, 62.4581) construction
  line L601 (24.8392, 62.4581) -> (24.83, 62.6207) construction
  line L602 (24.83, 62.6207) -> (24.8199, 62.7835) construction
  line L603 (24.8199, 62.7835) -> (24.8088, 62.9464) construction
  line L604 (24.8088, 62.9464) -> (24.7967, 63.1095) construction
  line L605 (24.7967, 63.1095) -> (24.7838, 63.2727) construction
  line L606 (24.7838, 63.2727) -> (24.77, 63.436) construction
  line L607 (24.77, 63.436) -> (24.7552, 63.5995) construction
  line L608 (24.7552, 63.5995) -> (24.7396, 63.7631) construction
  line L609 (24.7396, 63.7631) -> (24.723, 63.9268) construction
  line L610 (24.723, 63.9268) -> (24.7056, 64.0906) construction
  line L611 (24.7056, 64.0906) -> (24.6873, 64.2545) construction
  line L612 (24.6873, 64.2545) -> (24.6681, 64.4185) construction
  line L613 (24.6681, 64.4185) -> (24.648, 64.5826) construction
  line L614 (24.648, 64.5826) -> (24.6271, 64.7468) construction
  line L615 (24.6271, 64.7468) -> (24.6054, 64.9111) construction
  line L616 (24.6054, 64.9111) -> (24.5828, 65.0755) construction
  line L617 (24.5828, 65.0755) -> (24.5593, 65.24) construction
  line L618 (24.5593, 65.24) -> (24.535, 65.4046) construction
  line L619 (24.535, 65.4046) -> (24.5098, 65.5692) construction
  line L620 (24.5098, 65.5692) -> (24.4839, 65.734) construction
  line L621 (24.4839, 65.734) -> (24.4571, 65.8987) construction
  line L622 (24.4571, 65.8987) -> (24.4294, 66.0636) construction
  line L623 (24.4294, 66.0636) -> (24.401, 66.2285) construction
  line L624 (24.401, 66.2285) -> (24.3718, 66.3935) construction
  line L625 (24.3718, 66.3935) -> (24.3417, 66.5585) construction
  line L626 (24.3417, 66.5585) -> (24.3108, 66.7236) construction
  line L627 (24.3108, 66.7236) -> (24.2792, 66.8887) construction
  line L628 (24.2792, 66.8887) -> (24.2532, 67.0208) construction
  line L629 (24.2532, 67.0208) -> (24.2334, 67.1199) construction
  line L630 (24.2334, 67.1199) -> (24.22, 67.186) construction
  line L631 (24.22, 67.186) -> (24.2132, 67.2191) construction
  line L632 (31.1115, 52.5103) -> (31.1272, 52.5368) construction
  line L633 (31.1272, 52.5368) -> (31.1594, 52.5895) construction
  line L634 (31.1594, 52.5895) -> (31.2097, 52.6672) construction
  line L635 (31.2097, 52.6672) -> (31.2807, 52.7681) construction
  line L636 (31.2807, 52.7681) -> (31.3748, 52.8906) construction
  line L637 (31.3748, 52.8906) -> (31.4727, 53.0106) construction
  line L638 (31.4727, 53.0106) -> (31.5729, 53.1289) construction
  line L639 (31.5729, 53.1289) -> (31.6744, 53.2464) construction
  line L640 (31.6744, 53.2464) -> (31.7767, 53.3634) construction
  line L641 (31.7767, 53.3634) -> (31.88, 53.4797) construction
  line L642 (31.88, 53.4797) -> (31.9844, 53.5951) construction
  line L643 (31.9844, 53.5951) -> (32.0903, 53.7094) construction
  line L644 (32.0903, 53.7094) -> (32.1981, 53.8224) construction
  line L645 (32.1981, 53.8224) -> (32.3077, 53.934) construction
  line L646 (32.3077, 53.934) -> (32.419, 54.0444) construction
  line L647 (32.419, 54.0444) -> (32.5316, 54.1537) construction
  line L648 (32.5316, 54.1537) -> (32.6455, 54.2622) construction
  line L649 (32.6455, 54.2622) -> (32.7603, 54.3698) construction
  line L650 (32.7603, 54.3698) -> (32.876, 54.4767) construction
  line L651 (32.876, 54.4767) -> (32.9927, 54.5828) construction
  line L652 (32.9927, 54.5828) -> (33.1105, 54.6881) construction
  line L653 (33.1105, 54.6881) -> (33.2292, 54.7926) construction
  line L654 (33.2292, 54.7926) -> (33.3491, 54.8961) construction
  line L655 (33.3491, 54.8961) -> (33.47, 54.9988) construction
  line L656 (33.47, 54.9988) -> (33.5919, 55.1007) construction
  line L657 (33.5919, 55.1007) -> (33.7148, 55.2017) construction
  line L658 (33.7148, 55.2017) -> (33.8386, 55.302) construction
  line L659 (33.8386, 55.302) -> (33.9633, 55.4015) construction
  line L660 (33.9633, 55.4015) -> (34.0888, 55.5003) construction
  line L661 (34.0888, 55.5003) -> (34.2151, 55.5984) construction
  line L662 (34.2151, 55.5984) -> (34.3423, 55.6957) construction
  line L663 (34.3423, 55.6957) -> (34.4703, 55.7923) construction
  line L664 (34.4703, 55.7923) -> (34.5991, 55.8881) construction
  line L665 (34.5991, 55.8881) -> (34.7288, 55.9832) construction
  line L666 (34.7288, 55.9832) -> (34.8592, 56.0776) construction
  line L667 (34.8592, 56.0776) -> (34.9905, 56.1712) construction
  line L668 (34.9905, 56.1712) -> (35.1224, 56.2642) construction
  line L669 (35.1224, 56.2642) -> (35.2552, 56.3564) construction
  line L670 (35.2552, 56.3564) -> (35.3886, 56.448) construction
  line L671 (35.3886, 56.448) -> (35.5228, 56.5388) construction
  line L672 (35.5228, 56.5388) -> (35.6577, 56.629) construction
  line L673 (35.6577, 56.629) -> (35.7933, 56.7185) construction
  line L674 (35.7933, 56.7185) -> (35.9295, 56.8073) construction
  line L675 (35.9295, 56.8073) -> (36.0665, 56.8955) construction
  line L676 (36.0665, 56.8955) -> (36.2042, 56.9829) construction
  line L677 (36.2042, 56.9829) -> (36.3425, 57.0697) construction
  line L678 (36.3425, 57.0697) -> (36.4815, 57.1558) construction
  line L679 (36.4815, 57.1558) -> (36.6211, 57.2413) construction
  line L680 (36.6211, 57.2413) -> (36.7614, 57.3261) construction
  line L681 (36.7614, 57.3261) -> (36.9023, 57.4102) construction
  line L682 (36.9023, 57.4102) -> (37.0438, 57.4937) construction
  line L683 (37.0438, 57.4937) -> (37.186, 57.5765) construction
  line L684 (37.186, 57.5765) -> (37.3288, 57.6587) construction
  line L685 (37.3288, 57.6587) -> (37.4721, 57.7403) construction
  line L686 (37.4721, 57.7403) -> (37.6161, 57.8212) construction
  line L687 (37.6161, 57.8212) -> (37.7607, 57.9014) construction
  line L688 (37.7607, 57.9014) -> (37.9058, 57.981) construction
  line L689 (37.9058, 57.981) -> (38.0515, 58.06) construction
  line L690 (38.0515, 58.06) -> (38.1978, 58.1383) construction
  line L691 (38.1978, 58.1383) -> (38.3447, 58.216) construction
  line L692 (38.3447, 58.216) -> (38.4921, 58.2931) construction
  line L693 (38.4921, 58.2931) -> (38.6401, 58.3695) construction
  line L694 (38.6401, 58.3695) -> (38.7886, 58.4453) construction
  line L695 (38.7886, 58.4453) -> (38.9377, 58.5205) construction
  line L696 (38.9377, 58.5205) -> (39.0873, 58.595) construction
  line L697 (39.0873, 58.595) -> (39.2374, 58.669) construction
  line L698 (39.2374, 58.669) -> (39.3881, 58.7423) construction
  line L699 (39.3881, 58.7423) -> (39.5393, 58.8149) construction
  line L700 (39.5393, 58.8149) -> (39.6909, 58.887) construction
  line L701 (39.6909, 58.887) -> (39.8431, 58.9584) construction
  line L702 (39.8431, 58.9584) -> (39.9653, 59.0151) construction
  line L703 (39.9653, 59.0151) -> (40.0572, 59.0573) construction
  line L704 (40.0572, 59.0573) -> (40.1185, 59.0853) construction
  line L705 (40.1185, 59.0853) -> (40.1492, 59.0993) construction
  line L706 (-24.1948, 56.0345) -> (-24.2071, 56.0628) construction
  line L707 (-24.2071, 56.0628) -> (-24.2308, 56.1198) construction
  line L708 (-24.2308, 56.1198) -> (-24.264, 56.2062) construction
  line L709 (-24.264, 56.2062) -> (-24.3039, 56.3229) construction
  line L710 (-24.3039, 56.3229) -> (-24.3478, 56.4711) construction
  line L711 (-24.3478, 56.4711) -> (-24.3873, 56.6208) construction
  line L712 (-24.3873, 56.6208) -> (-24.4241, 56.7714) construction
  line L713 (-24.4241, 56.7714) -> (-24.4595, 56.9226) construction
  line L714 (-24.4595, 56.9226) -> (-24.494, 57.0741) construction
  line L715 (-24.494, 57.0741) -> (-24.5274, 57.226) construction
  line L716 (-24.5274, 57.226) -> (-24.5594, 57.3783) construction
  line L717 (-24.5594, 57.3783) -> (-24.5896, 57.5312) construction
  line L718 (-24.5896, 57.5312) -> (-24.6176, 57.6848) construction
  line L719 (-24.6176, 57.6848) -> (-24.6435, 57.8391) construction
  line L720 (-24.6435, 57.8391) -> (-24.6674, 57.994) construction
  line L721 (-24.6674, 57.994) -> (-24.6897, 58.1494) construction
  line L722 (-24.6897, 58.1494) -> (-24.7105, 58.3052) construction
  line L723 (-24.7105, 58.3052) -> (-24.7301, 58.4614) construction
  line L724 (-24.7301, 58.4614) -> (-24.7485, 58.6179) construction
  line L725 (-24.7485, 58.6179) -> (-24.7658, 58.7747) construction
  line L726 (-24.7658, 58.7747) -> (-24.7818, 58.9318) construction
  line L727 (-24.7818, 58.9318) -> (-24.7965, 59.0893) construction
  line L728 (-24.7965, 59.0893) -> (-24.8098, 59.2471) construction
  line L729 (-24.8098, 59.2471) -> (-24.8218, 59.4053) construction
  line L730 (-24.8218, 59.4053) -> (-24.8325, 59.5638) construction
  line L731 (-24.8325, 59.5638) -> (-24.842, 59.7226) construction
  line L732 (-24.842, 59.7226) -> (-24.8504, 59.8817) construction
  line L733 (-24.8504, 59.8817) -> (-24.8577, 60.0411) construction
  line L734 (-24.8577, 60.0411) -> (-24.8638, 60.2007) construction
  line L735 (-24.8638, 60.2007) -> (-24.8689, 60.3605) construction
  line L736 (-24.8689, 60.3605) -> (-24.8729, 60.5206) construction
  line L737 (-24.8729, 60.5206) -> (-24.8757, 60.6809) construction
  line L738 (-24.8757, 60.6809) -> (-24.8776, 60.8415) construction
  line L739 (-24.8776, 60.8415) -> (-24.8783, 61.0023) construction
  line L740 (-24.8783, 61.0023) -> (-24.878, 61.1633) construction
  line L741 (-24.878, 61.1633) -> (-24.8766, 61.3245) construction
  line L742 (-24.8766, 61.3245) -> (-24.8742, 61.4859) construction
  line L743 (-24.8742, 61.4859) -> (-24.8708, 61.6475) construction
  line L744 (-24.8708, 61.6475) -> (-24.8665, 61.8093) construction
  line L745 (-24.8665, 61.8093) -> (-24.8611, 61.9712) construction
  line L746 (-24.8611, 61.9712) -> (-24.8548, 62.1334) construction
  line L747 (-24.8548, 62.1334) -> (-24.8475, 62.2957) construction
  line L748 (-24.8475, 62.2957) -> (-24.8392, 62.4581) construction